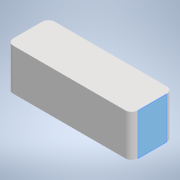
# Autodesk Inventor part: batt
Saved by Autodesk Inventor 2020 (Build 240168000, 168)
## iProperties
Created: 2022-12-14
Part Number: batt
Material: Generic
Document SubType Name: Modeling
Designer: Manish
Density: 1 g/cm^3
Appearance: Default
Author: Manish
Autodesk Inventor part; units mm, degrees
ref_plane "YZ Plane" through (0, 0, 0) normal (1, 0, 0) x (0, 1, 0)
ref_plane "XZ Plane" through (0, 0, 0) normal (0, 1, 0) x (-1, 0, 0)
ref_plane "XY Plane" through (0, 0, 0) normal (0, 0, 1) x (1, 0, 0)
sketch "Sketch1" plane through (0, 0, 0) normal (0, 1, 0) x (-1, 0, 0)
  line L0 (-6, 0) -> (-114, 0)
  line L1 (-120, -6) -> (-120, -34)
  line L2 (-114, -40) -> (-6, -40)
  line L3 (0, -34) -> (0, -6)
  line L4 (0, 0) -> (108, 0) construction
  arc A0 (0, -6) -> (-6, 0) centre (-6, -6) ccw
  arc A1 (-6, -40) -> (0, -34) centre (-6, -34) ccw
  arc A2 (-120, -34) -> (-114, -40) centre (-114, -34) ccw
  arc A3 (-114, 0) -> (-120, -6) centre (-114, -6) ccw
  point P0 (-120, 0)
  point P1 (-120, -40)
  dimension "d0" = 120
  dimension "d1" = 180
  dimension "d2" = 40
  dimension "d3" = 6
  constraints: 10 end point, 8 point on circle, 8 tangent, 6 point on line, 4 centre point, 3 equal radius, 2 horizontal, 2 parallel, 1 collinear, 1 perpendicular
  measures "d0" distance of L4.start point (-120, 0)
  measures "d1" angle of L0 L4
  measures "d2" distance of point (-120, -40) point (-120, 0)
  measures "d3" radius of A0
extrude "Extrusion1" add sketch "Sketch1" along normal blind 40
body "Solid1"
